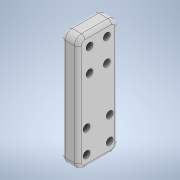
# Autodesk Inventor part: EboxTslotMountV2
Saved by Autodesk Inventor 2022 (Build 260153000, 153)
## iProperties
Created: 2022-02-26
Part Number: EboxTslotMountV2
Material: Generic
Document SubType Name: Modeling
Designer: Jorian Brusind
Density: 1 g/cm^3
Appearance: Default
Author: Jorian Brusind
Autodesk Inventor part; units mm, degrees
ref_plane "YZ Plane" through (0, 0, 0) normal (1, 0, 0) x (0, 1, 0)
ref_plane "XZ Plane" through (0, 0, 0) normal (0, 1, 0) x (-1, 0, 0)
ref_plane "XY Plane" through (0, 0, 0) normal (0, 0, 1) x (1, 0, 0)
sketch "Sketch1" plane through (0, 0, 0) normal (0, 1, 0) x (-1, 0, 0)
  line L0 (0, 0) -> (14, 0)
  line L1 (14, 0) -> (14, -35)
  line L2 (14, -35) -> (0, -35)
  line L3 (0, -35) -> (0, 0)
  dimension "d0" = 14
  dimension "d1" = 35
  constraints: 8 end point, 2 parallel, 1 horizontal, 1 perpendicular
  measures "d0" distance of L1.end L2.end
  measures "d1" distance of L0.end L1.end
extrude "Extrusion1" add sketch "Sketch1" along normal blind 100
sketch "Sketch2" plane through (0, 0, 0) normal (1, 0, 0) x (0, 0, -1)
  circle A0 centre (10, 90) radius 3
  line L0 (0, 0) -> (0, 100) projected
  line L1 (0, 100) -> (35, 100) projected
  circle A1 centre (25, 90) radius 3
  circle A2 centre (10, 70) radius 3
  circle A3 centre (25, 70) radius 3
  circle A4 centre (7.5, 10) radius 3
  line L2 (0, 0) -> (35, 0) projected
  circle A5 centre (27.5, 10) radius 3
  circle A6 centre (7.5, 30) radius 3
  circle A7 centre (27.5, 30) radius 3
  dimension "d4" = 6
  dimension "d5" = 10
  dimension "d6" = 10
  dimension "d9" = 15
  dimension "d12" = 20
  dimension "d15" = 6
  dimension "d16" = 10
  dimension "d17" = 7.5
  dimension "d20" = 20
  dimension "d23" = 20
  constraints: 8 centre point, 2 horizontal, 2 vertical, 12 other
  measures "d4" diameter of A0
  measures "d5" distance from line of L0 A0.centre
  measures "d6" distance from line of L1 A0.centre
  measures "d9" distance of A0.centre A1.centre
  measures "d12" distance of A0.centre A2.centre
  measures "d15" diameter of A4
  measures "d16" distance from line of L2 A4.centre
  measures "d17" distance from line of L0 A4.centre
  measures "d20" distance of A4.centre A5.centre
  measures "d23" distance of A4.centre A6.centre
extrude "Extrusion2" cut sketch "Sketch2" against normal through all
fillet "Fillet1" radius 6 4 edges at (-7, 0, 0) (-7, 0, -35) (-7, 100, 0) (-7, 100, -35)
fillet "Fillet2" radius 3 16 edges at (0, 98.2426, -33.2426) (0, 100, -17.5) (0, 98.2426, -1.7574) (0, 50, 0) (0, 1.7574, -1.7574) (0, 0, -17.5) (0, 1.7574, -33.2426) (0, 50, -35) (-14, 98.2426, -33.2426) (-14, 100, -17.5) (-14, 98.2426, -1.7574) (-14, 50, 0) (-14, 1.7574, -1.7574) (-14, 0, -17.5) (-14, 1.7574, -33.2426) (-14, 50, -35)
body "Solid1"
